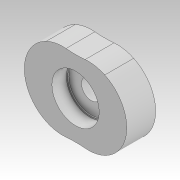
# Autodesk Inventor part: Rotor_NEW
Saved by Autodesk Inventor 2020 (Build 240168000, 168)
## iProperties
Created: 2022-01-30
Part Number: Rotor_NEW
Material: Generic
Document SubType Name: Modeling
Designer: DDeGo
Density: 1 g/cm^3
Appearance: Default
Author: DDeGo
Autodesk Inventor part; units mm, degrees
ref_plane "YZ Plane" through (0, 0, 0) normal (1, 0, 0) x (0, 1, 0)
ref_plane "XZ Plane" through (0, 0, 0) normal (0, 1, 0) x (-1, 0, 0)
ref_plane "XY Plane" through (0, 0, 0) normal (0, 0, 1) x (1, 0, 0)
sketch "Sketch1" plane through (0, 0, 0) normal (0, 0, 1) x (1, 0, 0)
  line L0 (4.8, 0) -> (-4.8, 0) construction
  line L1 (4.8, 14.7) -> (-4.8, 14.7) construction
  arc A0 (19.5, 0) -> (11.1318, 13.2664) centre (4.8, 0) ccw
  arc A1 (-4.8, 14.7) -> (-11.1318, 13.2664) centre (-4.8, 0) ccw construction
  line L2 (-19.5, 24.8831) -> (19.5, 24.8831) construction
  line L3 (19.5, 24.8831) -> (19.5, -24.8831) construction
  line L4 (19.5, -24.8831) -> (-19.5, -24.8831) construction
  line L5 (-19.5, -24.8831) -> (-19.5, 24.8831) construction
  line L6 (0, 0) -> (0, 14.7) construction
  arc A2 (-3.6434, 14.6131) -> (0, 14.45) centre (0, 55.2356) ccw
  arc A3 (-3.6434, 14.6131) -> (-11.1318, 13.2664) centre (-4.9297, 0.2718) ccw
  arc A4 (-11.1318, 13.2664) -> (-19.5, 0) centre (-4.8, 0) ccw
  arc A5 (0, 14.45) -> (3.6434, 14.6131) centre (0, 55.2356) ccw
  arc A6 (11.1318, 13.2664) -> (3.6434, 14.6131) centre (4.9297, 0.2718) ccw
  arc A7 (11.1318, 13.2664) -> (4.8, 14.7) centre (4.8, 0) ccw construction
  line L7 (-19.5, 0) -> (19.5, 0) construction
  arc A8 (11.1318, -13.2664) -> (19.5, 0) centre (4.8, 0) ccw
  arc A9 (0, -14.45) -> (-3.6434, -14.6131) centre (0, -55.2356) ccw
  arc A10 (-11.1318, -13.2664) -> (-3.6434, -14.6131) centre (-4.9297, -0.2718) ccw
  arc A11 (-19.5, 0) -> (-11.1318, -13.2664) centre (-4.8, 0) ccw
  arc A12 (3.6434, -14.6131) -> (0, -14.45) centre (0, -55.2356) ccw
  arc A13 (3.6434, -14.6131) -> (11.1318, -13.2664) centre (4.9297, -0.2718) ccw
  circle A14 centre (0, 0) radius 2.5
  line L8 (-11.1318, 13.2664) -> (0, 0) construction
  line L9 (-3.6434, 14.6131) -> (0, 0) construction
  dimension "d0" = 14.7
  dimension "d1" = 39
  dimension "d2" = 0.25
  dimension "d5" = 5
  dimension "d14" = 40
  dimension "d15" = 14
  constraints: 28 point on circle, 22 end point, 15 centre point, 12 tangent, 9 symmetric about line, 5 midpoint, 3 point on line, 2 equal radius, 2 horizontal, 2 parallel, 1 coincident, 1 perpendicular, 1 vertical, 6 other
  measures "d0" radius of A1
  measures "d1" distance of L2.start L2.end
  measures "d2" distance from line of L1 A2.end
  measures "d5" diameter of A14
  measures "d14" angle of L6 L8
  measures "d15" angle of L6 L9
extrude "Extrusion1" add sketch "Sketch1" along normal mid plane 11 contours A8 A13 A12 A9 A10 A11 A4 A3 A2 A5 A6 A0 | A14
sketch "Sketch2" plane through (0, 0, 0) normal (0, 1, 0) x (-1, 0, 0)
  line L0 (0, 0) -> (0, 5.5) construction
  line L1 (0, 5.5) -> (9, 5.5)
  line L2 (-3.6434, 5.5) -> (3.6434, 5.5) construction
  line L3 (3.6434, 5.5) -> (11.1318, 5.5) construction
  line L4 (11.1318, 5.5) -> (11.1318, 5.5) construction
  line L5 (11.1318, 5.5) -> (3.6434, 5.5) construction
  line L6 (3.6434, 5.5) -> (-3.6434, 5.5) construction
  line L7 (-3.6434, 5.5) -> (-11.1318, 5.5) construction
  line L8 (-11.1318, 5.5) -> (-11.1318, 5.5) construction
  line L9 (-11.1318, 5.5) -> (-3.6434, 5.5) construction
  line L10 (9, 5.5) -> (9, 0)
  line L11 (9, 0) -> (8.5, 0)
  line L12 (3.75, -0.5) -> (3.75, -5.5)
  line L13 (3.75, -5.5) -> (0, -5.5)
  line L14 (0, -5.5) -> (0, 5.5)
  line L15 (3.6434, -5.5) -> (-3.6434, -5.5) projected
  line L16 (-3.6434, -5.5) -> (-11.1318, -5.5) projected
  line L17 (-11.1318, -5.5) -> (-11.1318, -5.5) projected
  line L18 (-11.1318, -5.5) -> (-3.6434, -5.5) projected
  line L19 (-3.6434, -5.5) -> (3.6434, -5.5) projected
  line L20 (3.6434, -5.5) -> (11.1318, -5.5) projected
  line L21 (11.1318, -5.5) -> (11.1318, -5.5) projected
  line L22 (11.1318, -5.5) -> (3.6434, -5.5) projected
  line L23 (8.5, 0) -> (8.5, -0.5)
  line L24 (8.5, -0.5) -> (3.75, -0.5)
  dimension "d8" = 3.75
  dimension "d9" = 5.5
  dimension "d10" = 9
  dimension "d12" = 0.5
  dimension "d13" = 0.5
  constraints: 18 end point, 5 perpendicular, 2 midpoint, 2 vertical, 1 collinear, 1 horizontal, 1 point on line
  measures "d8" distance between parallel lines of L12 L14
  measures "d9" distance between parallel lines of L5 L11
  measures "d10" distance between parallel lines of L0 L10
  measures "d12" distance of L11.end L23.end
  measures "d13" distance of L10.end L11.end
revolve "Revolution1" cut sketch "Sketch2" angle 360 about axis through (0, 0, 0) along (0, 0, 1)
sketch "Sketch3" plane through (0, 0, -5.5) normal (0, 0, -1) x (-1, 0, 0)
  circle A0 centre (0, 0) radius 12.5
  circle A1 centre (0, 0) radius 3.75 projected
  dimension "d18" = 25
  constraints: 1 centre point, 1 coincident
  measures "d18" diameter of A0
extrude "Extrusion2" add sketch "Sketch3" along normal blind 10
spur gear teeth "Spur Gear1" teeth 16 pitch diameter 9.6 tip diameter 10.6669 root diameter 7.9669 face width 3 trims to tip circle yes start plane through (0, 0, -15.5) normal (0, 0, -1) x (-1, 0, 0)
ref_plane "Work Plane1" through (0, 0, -2) normal (0, 0, -1) x (-1, 0, 0)
sketch "Sketch4" plane through (0, 0, -12.5) normal (0, 0, -1) x (-1, 0, 0)
  arc A0 (3.9518, 3.5817) -> (3.5817, 3.9518) centre (0, 0) ccw projected
  arc A1 (3.1996, 2.3729) -> (3.9518, 3.5817) centre (-0.1257, 5.2809) ccw projected
  arc A2 (4.8214, 2.2804) -> (3.4167, 2.0479) centre (4.8308, -2.137) ccw projected
  arc A3 (5.0217, 1.7968) -> (4.8214, 2.2804) centre (0, 0) ccw projected
  arc A4 (3.8641, 0.9679) -> (5.0217, 1.7968) centre (1.9048, 4.927) ccw projected
  arc A5 (5.327, 0.2617) -> (3.9404, 0.5845) centre (3.6453, -3.823) ccw projected
  arc A6 (5.327, -0.2617) -> (5.327, 0.2617) centre (0, 0) ccw projected
  arc A7 (3.9404, -0.5845) -> (5.327, -0.2617) centre (3.6453, 3.823) ccw projected
  arc A8 (5.0217, -1.7968) -> (3.8641, -0.9679) centre (1.9048, -4.927) ccw projected
  arc A9 (4.8214, -2.2804) -> (5.0217, -1.7968) centre (0, 0) ccw projected
  arc A10 (3.4167, -2.0479) -> (4.8214, -2.2804) centre (4.8308, 2.137) ccw projected
  arc A11 (3.9518, -3.5817) -> (3.1996, -2.3729) centre (-0.1257, -5.2809) ccw projected
  arc A12 (3.5817, -3.9518) -> (3.9518, -3.5817) centre (0, 0) ccw projected
  arc A13 (2.3729, -3.1996) -> (3.5817, -3.9518) centre (5.2809, 0.1257) ccw projected
  arc A14 (2.2804, -4.8214) -> (2.0479, -3.4167) centre (-2.137, -4.8308) ccw projected
  arc A15 (1.7968, -5.0217) -> (2.2804, -4.8214) centre (0, 0) ccw projected
  arc A16 (0.9679, -3.8641) -> (1.7968, -5.0217) centre (4.927, -1.9048) ccw projected
  arc A17 (0.2617, -5.327) -> (0.5845, -3.9404) centre (-3.823, -3.6453) ccw projected
  arc A18 (-0.2617, -5.327) -> (0.2617, -5.327) centre (0, 0) ccw projected
  arc A19 (-0.5845, -3.9404) -> (-0.2617, -5.327) centre (3.823, -3.6453) ccw projected
  arc A20 (-1.7968, -5.0217) -> (-0.9679, -3.8641) centre (-4.927, -1.9048) ccw projected
  arc A21 (-2.2804, -4.8214) -> (-1.7968, -5.0217) centre (0, 0) ccw projected
  arc A22 (-2.0479, -3.4167) -> (-2.2804, -4.8214) centre (2.137, -4.8308) ccw projected
  arc A23 (-3.5817, -3.9518) -> (-2.3729, -3.1996) centre (-5.2809, 0.1257) ccw projected
  arc A24 (-3.9518, -3.5817) -> (-3.5817, -3.9518) centre (0, 0) ccw projected
  arc A25 (-3.1996, -2.3729) -> (-3.9518, -3.5817) centre (0.1257, -5.2809) ccw projected
  arc A26 (-4.8214, -2.2804) -> (-3.4167, -2.0479) centre (-4.8308, 2.137) ccw projected
  arc A27 (-5.0217, -1.7968) -> (-4.8214, -2.2804) centre (0, 0) ccw projected
  arc A28 (-3.8641, -0.9679) -> (-5.0217, -1.7968) centre (-1.9048, -4.927) ccw projected
  arc A29 (-5.327, -0.2617) -> (-3.9404, -0.5845) centre (-3.6453, 3.823) ccw projected
  arc A30 (-5.327, 0.2617) -> (-5.327, -0.2617) centre (0, 0) ccw projected
  arc A31 (-3.9404, 0.5845) -> (-5.327, 0.2617) centre (-3.6453, -3.823) ccw projected
  arc A32 (-5.0217, 1.7968) -> (-3.8641, 0.9679) centre (-1.9048, 4.927) ccw projected
  arc A33 (-4.8214, 2.2804) -> (-5.0217, 1.7968) centre (0, 0) ccw projected
  arc A34 (-3.4167, 2.0479) -> (-4.8214, 2.2804) centre (-4.8308, -2.137) ccw projected
  arc A35 (-3.9518, 3.5817) -> (-3.1996, 2.3729) centre (0.1257, 5.2809) ccw projected
  arc A36 (-3.5817, 3.9518) -> (-3.9518, 3.5817) centre (0, 0) ccw projected
  arc A37 (-2.3729, 3.1996) -> (-3.5817, 3.9518) centre (-5.2809, -0.1257) ccw projected
  arc A38 (-2.2804, 4.8214) -> (-2.0479, 3.4167) centre (2.137, 4.8308) ccw projected
  arc A39 (-1.7968, 5.0217) -> (-2.2804, 4.8214) centre (0, 0) ccw projected
  arc A40 (-0.9679, 3.8641) -> (-1.7968, 5.0217) centre (-4.927, 1.9048) ccw projected
  arc A41 (-0.2617, 5.327) -> (-0.5845, 3.9404) centre (3.823, 3.6453) ccw projected
  arc A42 (0.2617, 5.327) -> (-0.2617, 5.327) centre (0, 0) ccw projected
  arc A43 (0.5845, 3.9404) -> (0.2617, 5.327) centre (-3.823, 3.6453) ccw projected
  arc A44 (1.7968, 5.0217) -> (0.9679, 3.8641) centre (4.927, 1.9048) ccw projected
  arc A45 (2.2804, 4.8214) -> (1.7968, 5.0217) centre (0, 0) ccw projected
  arc A46 (2.0479, 3.4167) -> (2.2804, 4.8214) centre (-2.137, 4.8308) ccw projected
  arc A47 (3.5817, 3.9518) -> (2.3729, 3.1996) centre (5.2809, -0.1257) ccw projected
  circle A48 centre (0, 0) radius 12.5 projected
  arc A49 (3.4167, 2.0479) -> (3.1996, 2.3729) centre (0, 0) ccw projected
  arc A50 (3.9404, 0.5845) -> (3.8641, 0.9679) centre (0, 0) ccw projected
  arc A51 (3.8641, -0.9679) -> (3.9404, -0.5845) centre (0, 0) ccw projected
  arc A52 (3.1996, -2.3729) -> (3.4167, -2.0479) centre (0, 0) ccw projected
  arc A53 (2.0479, -3.4167) -> (2.3729, -3.1996) centre (0, 0) ccw projected
  arc A54 (0.5845, -3.9404) -> (0.9679, -3.8641) centre (0, 0) ccw projected
  arc A55 (-0.9679, -3.8641) -> (-0.5845, -3.9404) centre (0, 0) ccw projected
  arc A56 (-2.3729, -3.1996) -> (-2.0479, -3.4167) centre (0, 0) ccw projected
  arc A57 (-3.4167, -2.0479) -> (-3.1996, -2.3729) centre (0, 0) ccw projected
  arc A58 (-3.9404, -0.5845) -> (-3.8641, -0.9679) centre (0, 0) ccw projected
  arc A59 (-3.8641, 0.9679) -> (-3.9404, 0.5845) centre (0, 0) ccw projected
  arc A60 (-3.1996, 2.3729) -> (-3.4167, 2.0479) centre (0, 0) ccw projected
  arc A61 (-2.0479, 3.4167) -> (-2.3729, 3.1996) centre (0, 0) ccw projected
  arc A62 (-0.5845, 3.9404) -> (-0.9679, 3.8641) centre (0, 0) ccw projected
  arc A63 (0.9679, 3.8641) -> (0.5845, 3.9404) centre (0, 0) ccw projected
  arc A64 (2.3729, 3.1996) -> (2.0479, 3.4167) centre (0, 0) ccw projected
  point P0 (0, 0)
extrude "Extrusion3" cut sketch "Sketch4" against normal up to surface (10.5 mm away)
ref_plane "Work Plane2" through (0, 0, -5.25) normal (0, 0, -1) x (-1, 0, 0)
sketch "Sketch5" plane through (0, 0, -15.5) normal (0, 0, -1) x (-1, 0, 0)
  circle A0 centre (0, 0) radius 7.9397
  constraints: 1 centre point, 1 coincident
extrude "Extrusion4" cut sketch "Sketch5" against normal up to surface (10.25 mm away)
fillet "Fillet1" radius 0.3 32 edges at (-1.7968, -5.0217, -3.625) (-2.2804, -4.8214, -3.625) (-3.5817, -3.9518, -3.625) (-3.9518, -3.5817, -3.625) (-5.0217, -1.7968, -3.625) (-4.8214, -2.2804, -3.625) (-5.327, -0.2617, -3.625) (-5.327, 0.2617, -3.625) (-5.0217, 1.7968, -3.625) (-4.8214, 2.2804, -3.625) (-3.9518, 3.5817, -3.625) (-3.5817, 3.9518, -3.625) (-2.2804, 4.8214, -3.625) (-1.7968, 5.0217, -3.625) (-0.2617, 5.327, -3.625) (0.2617, 5.327, -3.625) (2.2804, 4.8214, -3.625) (1.7968, 5.0217, -3.625) (3.5817, 3.9518, -3.625) (3.9518, 3.5817, -3.625) (4.8214, 2.2804, -3.625) (5.0217, 1.7968, -3.625) (5.327, 0.2617, -3.625) (5.327, -0.2617, -3.625) (5.0217, -1.7968, -3.625) (4.8214, -2.2804, -3.625) (3.9518, -3.5817, -3.625) (3.5817, -3.9518, -3.625) (2.2804, -4.8214, -3.625) (1.7968, -5.0217, -3.625) (0.2617, -5.327, -3.625) (-0.2617, -5.327, -3.625)
body "Solid1"
